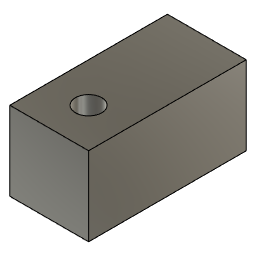
Wall_E_STANDOFF_TOP v1 (Autodesk Fusion 360 design; units mm, degrees)
Autodesk Fusion 360 part; units mm, degrees
note: some values were not read from the file. Set by a fixed rule: which sketch regions a step uses.
sketch "Sketch1" plane through (0, 0, 0) normal (0, 1, 0) x (1, 0, 0)
  line L0 (0, 0) -> (15, 0)
  line L1 (15, 0) -> (15, -15)
  line L2 (15, -15) -> (0, -15)
  line L3 (0, -15) -> (0, 0)
  dimension "d1" = 15
  dimension "d2" = 15
  constraint horizontal L0
  constraint vertical L1
  constraint horizontal L2
  constraint vertical L3
  constraint coincident L0.start L3.end
  measures "d1" distance of L0.start L0.end
  measures "d2" distance of L0.start L2.end
extrude "Extrude1" add sketch "Sketch1" along normal blind 30
sketch "Sketch3" plane through (0, 0, 15) normal (0, 0, 1) x (-1, 0, 0)
  line L0 (0, 0) -> (-15, 0)
  line L1 (-15, 0) -> (-15, -30)
  line L2 (-15, -30) -> (0, -30)
  line L3 (0, -30) -> (0, 0)
  line L4 (0, 0) -> (-9.4343, 0)
  line L5 (-9.4343, 0) -> (-9.4343, -2.5)
  line L6 (-9.4343, -2.5) -> (0, -2.5)
  line L7 (0, -2.5) -> (0, 0)
  line L8 (0, 0) -> (-7.5, 0)
  line L9 (-7.5, 0) -> (-7.5, -11.3998)
  line L10 (-7.5, -11.3998) -> (-7.5, -2.5)
  line L11 (-7.5, -2.5) -> (-7.5, -7.5)
  circle A0 centre (-7.5, -7.5) radius 2.5
  dimension "d13" = 2.5
  dimension "d14" = 5
  dimension "d15" = 5
  constraint horizontal L4
  constraint vertical L5
  constraint horizontal L6
  constraint vertical L7
  constraint coincident L0.start L3.end
  constraint midpoint L0 L8.end
  constraint perpendicular L6 L9
  constraint coincident L9 L10.end
  constraint coincident L6 L10.end
  constraint perpendicular L6 L11
  constraint coincident L11.end A0.centre
  measures "d13" distance of L0.start L6.end
  measures "d14" distance of L10.end L11.end
  measures "d15" diameter of A0
extrude "Extrude3" cut sketch "Sketch3" against normal blind 34 contours L9 L10 L11 A0 | L9 L10 L11 A0
